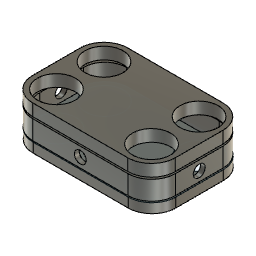
UAV v3 (Autodesk Fusion 360 design; units mm, degrees)
Autodesk Fusion 360 part; units mm, degrees
sketch "Sketch1" plane through (0, 0, 0) normal (0, 0, 1) x (1, 0, 0)
  line L0 (-100, 100) -> (100, 100)
  line L1 (150, 50) -> (150, -50)
  line L2 (100, -100) -> (-100, -100)
  line L3 (-150, -50) -> (-150, 50)
  arc A0 (-100, 100) -> (-150, 50) centre (-100, 50) ccw
  arc A1 (150, 50) -> (100, 100) centre (100, 50) ccw
  arc A2 (100, -100) -> (150, -50) centre (100, -50) ccw
  arc A3 (-150, -50) -> (-100, -100) centre (-100, -50) ccw
  circle A4 centre (-100, 50) radius 40
  circle A5 centre (100, 50) radius 40
  circle A6 centre (-100, -50) radius 40
  circle A7 centre (100, -50) radius 40
  dimension "d1" = 50
  dimension "d2" = 50
  dimension "d3" = 50
  constraint horizontal L0
  constraint vertical L1
  constraint horizontal L2
  constraint vertical L3
  constraint tangent L0 A0
  constraint tangent L3 A0
  constraint tangent L0 A1
  constraint tangent L1 A1
  constraint tangent L1 A2
  constraint tangent L2 A2
  constraint tangent L2 A3
  constraint tangent L3 A3
  constraint equal A2 A3
  constraint concentric A0 A4
  constraint concentric A1 A5
  constraint concentric A3 A6
  constraint concentric A2 A7
  measures "d1" radius of A0
  measures "d2" radius of A1
  measures "d3" radius of A2
extrude "Extrude1" add sketch "Sketch1" along normal blind 20 makes body 1
sketch "Sketch2" plane through (0, 0, 20) normal (0, 0, 1) x (-1, 0, 0)
  circle A0 centre (-100, -50) radius 40
  circle A1 centre (-100, 50) radius 40
  circle A2 centre (100, 50) radius 40
  circle A3 centre (100, -50) radius 40
  arc A4 (100, -100) -> (150, -50) centre (100, -50) ccw
  line L0 (150, -50) -> (150, 50)
  arc A5 (150, 50) -> (100, 100) centre (100, 50) ccw
  line L1 (100, 100) -> (-100, 100)
  arc A6 (-100, 100) -> (-150, 50) centre (-100, 50) ccw
  line L2 (-150, 50) -> (-150, -50)
  arc A7 (-150, -50) -> (-100, -100) centre (-100, -50) ccw
  line L3 (-100, -100) -> (100, -100)
sketch "Sketch3" plane through (0, 0, 20) normal (0, 0, 1) x (-1, 0, 0)
  line L0 (-100, -150) -> (100, -150)
  line L1 (150, -200) -> (150, -300)
  line L2 (100, -350) -> (-100, -350)
  line L3 (-150, -300) -> (-150, -200)
  arc A0 (-100, -150) -> (-150, -200) centre (-100, -200) ccw
  arc A1 (150, -200) -> (100, -150) centre (100, -200) ccw
  arc A2 (100, -350) -> (150, -300) centre (100, -300) ccw
  arc A3 (-150, -300) -> (-100, -350) centre (-100, -300) ccw
  circle A4 centre (-100, -200) radius 40
  circle A5 centre (100, -200) radius 40
  circle A6 centre (-100, -300) radius 40
  circle A7 centre (100, -300) radius 40
  dimension "d6" = 50
  dimension "d7" = 80
  dimension "d8" = 80
  dimension "d9" = 80
  dimension "d10" = 80
  constraint horizontal L0
  constraint vertical L1
  constraint horizontal L2
  constraint vertical L3
  constraint tangent L0 A0
  constraint tangent L3 A0
  constraint tangent L0 A1
  constraint tangent L1 A1
  constraint equal A0 A1
  constraint tangent L1 A2
  constraint tangent L2 A2
  constraint equal A0 A2
  constraint tangent L2 A3
  constraint tangent L3 A3
  constraint equal A0 A3
  constraint concentric A0 A4
  constraint concentric A1 A5
  constraint concentric A3 A6
  constraint concentric A2 A7
  measures "d6" radius of A0
  measures "d7" diameter of A4
  measures "d8" diameter of A5
  measures "d9" diameter of A6
  measures "d10" diameter of A7
extrude "Extrude2" add sketch "Sketch3" along normal blind 25 separate body makes body 2
move_body "Move1" bodies 2 to x (1, 0, 0) y (0, 1, 0) z (0, 0, 1) at (0, -247.6259, 40.7159)
move_body "Move2" bodies 2 to x (1, 0, 0) y (0, 1, 0) z (0, 0, 1) at (0, 273.4303, -52.2928)
move_body "Move3" bodies 2 to x (1, 0, 0) y (0, 1, 0) z (0, 0, 1) at (0, -278.3475, 44.9709)
sketch "Sketch4" plane through (0, 0, 78.394) normal (0, 0, 1) x (-1, 0, 0)
  circle A0 centre (100, -47.4569) radius 40
  circle A1 centre (100, 52.5431) radius 40
  circle A2 centre (-100, -47.4569) radius 40
  circle A3 centre (-100, 52.5431) radius 40
  arc A4 (-100, 102.5431) -> (-150, 52.5431) centre (-100, 52.5431) ccw
  line L0 (-150, 52.5431) -> (-150, -47.4569)
  arc A5 (-150, -47.4569) -> (-100, -97.4569) centre (-100, -47.4569) ccw
  line L1 (-100, -97.4569) -> (100, -97.4569)
  arc A6 (100, -97.4569) -> (150, -47.4569) centre (100, -47.4569) ccw
  line L2 (150, -47.4569) -> (150, 52.5431)
  arc A7 (150, 52.5431) -> (100, 102.5431) centre (100, 52.5431) ccw
  line L3 (100, 102.5431) -> (-100, 102.5431)
  line L4 (100, 150) -> (-100, 150)
  line L5 (-150, 200) -> (-150, 300)
  line L6 (-100, 350) -> (100, 350)
  line L7 (150, 300) -> (150, 200)
  arc A8 (100, 150) -> (150, 200) centre (100, 200) ccw
  arc A9 (-150, 200) -> (-100, 150) centre (-100, 200) ccw
  arc A10 (150, 300) -> (100, 350) centre (100, 300) ccw
  arc A11 (-100, 350) -> (-150, 300) centre (-100, 300) ccw
  line L8 (-100.2388, 157.9963) -> (95.1857, 157.9963)
  line L9 (140.1857, 202.9963) -> (140.1857, 295)
  line L10 (95.1857, 340) -> (-100.2388, 340)
  line L11 (-140.2388, 300) -> (-140.2388, 197.9963)
  arc A12 (95.1857, 157.9963) -> (140.1857, 202.9963) centre (95.1857, 202.9963) ccw
  arc A13 (140.1857, 295) -> (95.1857, 340) centre (95.1857, 295) ccw
  arc A14 (-140.2388, 197.9963) -> (-100.2388, 157.9963) centre (-100.2388, 197.9963) ccw
  arc A15 (-100.2388, 340) -> (-140.2388, 300) centre (-100.2388, 300) ccw
  dimension "d13" = 50
  dimension "d14" = 45
  dimension "d15" = 40
  constraint horizontal L4
  constraint vertical L5
  constraint horizontal L6
  constraint vertical L7
  constraint tangent L4 A8
  constraint tangent L7 A8
  constraint tangent L4 A9
  constraint tangent L5 A9
  constraint equal A8 A9
  constraint tangent L6 A10
  constraint tangent L7 A10
  constraint equal A8 A10
  constraint tangent L5 A11
  constraint tangent L6 A11
  constraint equal A8 A11
  constraint horizontal L8
  constraint vertical L9
  constraint horizontal L10
  constraint vertical L11
  constraint tangent L8 A12
  constraint tangent L9 A12
  constraint tangent L9 A13
  constraint tangent L10 A13
  constraint equal A12 A13
  constraint tangent L8 A14
  constraint tangent L11 A14
  constraint tangent L10 A15
  constraint tangent L11 A15
  constraint equal A14 A15
  measures "d13" radius of A8
  measures "d14" radius of A12
  measures "d15" radius of A14
extrude "Extrude3" add sketch "Sketch4" along normal blind 40 separate body contours L4 L5 L6 L7 A8 A9 A10 A11 makes body 3
move_body "Move4" bodies 2 to x (1, 0, 0) y (0, 1, 0) z (0, 0, 1) at (-300.9267, 264.9611, -247.7216)
move_body "Move5" bodies 3 to x (1, 0, 0) y (0, 1, 0) z (0, 0, 1) at (-50.6838, 244.6089, -4.5449)
move_body "Move6" bodies 3 to x (1, 0, 0) y (0, 1, 0) z (0, 0, 1) at (50, 0, -50)
move_body "Move7" bodies 2 to x (1, 0, 0) y (0, 1, 0) z (0, 0, 1) at (0, 0, 250)
move_body "Move8" bodies 3 to x (1, 0, 0) y (0, 1, 0) z (0, 0, 1) at (0, 5.3408, -1.526)
hole "Hole1" at (149.3162, -0.0503, 42.3231) direction (-1, 0, 0) diameter 25 depth 25 tip angle 118 bodies 3
hole "Hole2" at (-150.6838, -0.0503, 42.3231) direction (1, 0, 0) diameter 25 depth 25 tip angle 118 bodies 3
hole "Hole3" at (-0.6838, -100.0503, 42.3231) direction (0, 1, 0) diameter 25 depth 75 tip angle 118 bodies 3
hole "Hole4" at (-0.6838, 99.9497, 42.3231) direction (0, -1, 0) diameter 25 depth 75 tip angle 118 bodies 3
move_body "Move9" bodies 2 to x (1, 0, 0) y (0, 1, 0) z (0, 0, 1) at (299.9757, -262.4359, 10.37)
